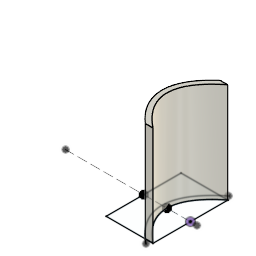
Single Curve Rectangular Reflector v2 (Autodesk Fusion 360 design; units mm, degrees)
Autodesk Fusion 360 part; units mm, degrees
sketch "Sketch1" plane through (0, 0, 0) normal (0, 0, 1) x (1, 0, 0)
  line L0 (0, 75) -> (-93.75, 75)
  line L1 (-93.75, 75) -> (-93.75, -75)
  line L2 (-93.75, -75) -> (0, -75)
  line L3 (0, -75) -> (0, 75)
  line L4 (0, 0) -> (-250, 0) construction
  spline S0 degree 2 poles (0, -75) (-93.75, 0) (0, 75) knots 0 0 0 17.688715 17.688715 17.688715
  spline S1 degree 3 poles (-6.247, -82.8087) (-22.5068, -69.8008) (-35.0297, -56.5704) (-43.6362, -42.8) (-49.9938, -32.6279) (-54.1945, -22.1238) (-55.9441, -11.4108) (-57.7012, -0.6518) (-56.9391, 10.2664) (-53.746, 20.8975) (-50.2745, 32.456) (-44.0021, 43.6588) (-35.2519, 54.5359) (-27.5183, 64.1492) (-17.8379, 73.5359) (-6.247, 82.8087) knots 0 0 0 0 4.422179 4.422179 4.422179 7.688813 7.688813 7.688813 10.969476 10.969476 10.969476 14.536327 14.536327 14.536327 17.688715 17.688715 17.688715 17.688715
  point P0 (13.125, 0)
  point P1 (-46.875, 0)
  constraint horizontal L0
  constraint vertical L1
  constraint horizontal L2
  constraint vertical L3
  constraint midpoint L4.start L3
  constraint coincident L4.start origin
  constraint perpendicular L3 L4
  constraint coincident S0 P1
  constraint coincident L4 P1
  constraint collinear L4.start P0 P1
extrude "Extrude2" add sketch "Sketch1" along normal blind 200 contours L0 L2 S0 S1
extrude "Extrude1" [suppressed]
equation "Focal = 0.06 m"
equation "Radius = 0.15 m"
equation "Hight = 0.20 m"
equation "d8 = Hight"
equation "d13 = Radius"
equation "d14 = ( Radius ^ 2 ) / ( 4 * Focal )"
equation "d17 = Focal"
equation "d18 = Hight"
